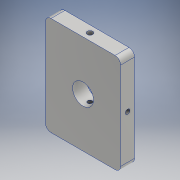
# Autodesk Inventor part: CardMount_sjc
Saved by Autodesk Inventor 2017 SP1 (Build 210196100, 196)
## iProperties
Created: 2017-04-07
Part Number: CardMount_sjc
Material: Generic
Document SubType Name: Modeling
Designer: Sam
Density: 1 g/cm^3
Appearance: Aluminum - Flat
Author: Sam
Revision Number: ANY
Autodesk Inventor part; units mm, degrees
ref_plane "YZ Plane" through (0, 0, 0) normal (1, 0, 0) x (0, 1, 0)
ref_plane "XZ Plane" through (0, 0, 0) normal (0, 1, 0) x (-1, 0, 0)
ref_plane "XY Plane" through (0, 0, 0) normal (0, 0, 1) x (1, 0, 0)
sketch "Sketch9" plane through (0, 0, 0) normal (0, 1, 0) x (-1, 0, 0)
  line L0 (-27, 35.5) -> (27, 35.5)
  line L1 (27, 35.5) -> (27, -35.5)
  line L2 (27, -35.5) -> (-27, -35.5)
  line L3 (-27, -35.5) -> (-27, 35.5)
  line L4 (-27, 35.5) -> (27, -35.5) construction
  line L5 (27, 35.5) -> (-27, -35.5) construction
  point P0 (0, 0)
  dimension "d39" = 54
  dimension "d40" = 71
  constraints: 12 end point, 2 midpoint, 2 parallel, 1 horizontal, 1 perpendicular
  measures "d39" distance of L1.end L2.end
  measures "d40" distance of L0.end L1.end
extrude "Extrusion4" add sketch "Sketch9" along normal blind 10
sketch "Sketch10" plane through (0, 10, 0) normal (0, 1, 0) x (1, 0, 0)
  circle A0 centre (0, 0) radius 7.5
  dimension "d43" = 15
  constraints: 1 centre point, 1 coincident
  measures "d43" diameter of A0
extrude "Extrusion5" cut sketch "Sketch10" against normal blind 10
sketch "Sketch11" plane through (27, 0, 35.5) normal (1, 0, 0) x (0, 0, -1)
  point P0 (35.5, 0)
  point P1 (35.5, 5)
hole "Hole5" at (27, 5, 0) direction (-1, 0, 0) diameter 3.242 depth 11.8 tip angle 118 thread size "M4x0.7" class "6H" standard "ANSI Metric M Profile"
sketch "Sketch12" plane through (0, 10, 0) normal (0, 1, 0) x (1, 0, 0)
  point P0 (0, 0)
sketch "Sketch13" plane through (0, 10, 0) normal (0, 1, 0) x (1, 0, 0)
  point P0 (0, 0)
  point P1 (22.809, -31.309)
  point P2 (-22.809, 31.309)
  point P3 (-22.809, -31.309)
  point P4 (22.809, 31.309)
hole "Hole6" at (-22.809, 10, 31.309) at (-22.809, 10, -31.309) at (22.809, 10, -31.309) at (22.809, 10, 31.309) direction (0, -1, 0) diameter 2.459 depth 8.8 tip angle 118 thread size "M3x0.5" class "6H" standard "ANSI Metric M Profile"
fillet "Fillet3" radius 4 4 edges at (-27, 5, -35.5) (-27, 5, 35.5) (27, 5, -35.5) (27, 5, 35.5)
sketch "Sketch14" plane through (23, 0, -35.5) normal (0, 0, -1) x (-1, 0, 0)
  point P0 (23, 0)
  point P1 (23, 5)
sketch "Sketch15" plane through (-23, 0, 35.5) normal (0, 0, 1) x (1, 0, 0)
  point P0 (23, 0)
  point P1 (23, 5)
hole "Hole7" at (0, 5, 35.5) direction (0, 0, -1) diameter 4 depth 20
hole "Hole8" at (0, 5, -35.5) direction (0, 0, 1) diameter 4 depth 20
sketch "Sketch16" plane through (0, 5, 15.5) normal (0, 0, 1) x (1, 0, 0)
  point P0 (0, -5)
  point P1 (0, 0)
sketch "Sketch17" plane through (0, 5, -15.5) normal (0, 0, -1) x (-1, 0, 0)
  point P0 (0, -5)
  point P1 (0, 0)
hole "Hole9" at (0, 5, -15.5) direction (0, 0, 1) diameter 3.242 depth 11.8 thread size "M4x0.7" class "6H" standard "ANSI Metric M Profile"
hole "Hole10" at (0, 5, 15.5) direction (0, 0, -1) diameter 3.242 depth 11.8 thread size "M4x0.7" class "6H" standard "ANSI Metric M Profile"
equation "\"z\" = 71"
equation "\"x\" = 54"
equation "\"corner\" = 4"
body "Solid2"
